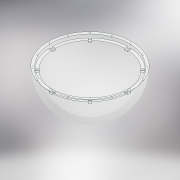
# Autodesk Inventor part: Bol
Saved by Autodesk Inventor 2022 (Build 260153000, 153)
## iProperties
Created: 2022-03-08
Part Number: Bol
Material: Glass
Document SubType Name: Modeling
Designer: 32497
Density: 2.18 g/cm^3
Appearance: Clear
Author: 32497
Autodesk Inventor part; units mm, degrees
ref_plane "YZ Plane" through (0, 0, 0) normal (1, 0, 0) x (0, 1, 0)
ref_plane "XZ Plane" through (0, 0, 0) normal (0, 1, 0) x (-1, 0, 0)
ref_plane "XY Plane" through (0, 0, 0) normal (0, 0, 1) x (1, 0, 0)
sketch "Sketch1" plane through (0, 0, 0) normal (0, 1, 0) x (-1, 0, 0)
  arc A0 (0, 150) -> (0, -150) centre (0, 0) ccw
  arc A1 (0, 130) -> (0, -130) centre (0, 0) ccw
  line L0 (0, -150) -> (0, 150)
  line L1 (150, 0) -> (-150, 0)
  circle A2 centre (0, 0) radius 141
  dimension "d0" = 300
  dimension "d1" = 260
  dimension "d9" = 282
  constraints: 5 point on circle, 4 end point, 3 centre point, 3 coincident, 2 point on line, 1 vertical
  measures "d0" diameter of A0
  measures "d1" diameter of A1
  measures "d9" diameter of A2
revolve "Revolution1" add sketch "Sketch1" angle 180 about axis through (0, 0, -150) along (0, 0, -1) contours L0 A2 L1 A0 | L1 A2 L0 A0 | L0 A1 L1 A2 | L1 A1 L0 A2
sketch "Sketch6" plane through (0, 0, 0) normal (0, 1, 0) x (1, 0, 0)
  circle A0 centre (0, 0) radius 140
  circle A1 centre (0, 0) radius 128.5
  dimension "d19" = 280
  dimension "d20" = 257
  constraints: 2 centre point, 2 coincident
  measures "d19" diameter of A0
  measures "d20" diameter of A1
extrude "Extrusion3" cut sketch "Sketch6" against normal blind 12.5
sketch "Sketch7" plane through (0, -12.5, 0) normal (0, 1, 0) x (1, 0, 0)
  line L0 (-5, 140.4975) -> (5, 140.4975)
  line L1 (5, 140.4975) -> (5, 128.8975)
  line L2 (5, 128.8975) -> (-5, 128.8975)
  line L3 (-5, 128.8975) -> (-5, 140.4975)
  circle A0 centre (0, 0) radius 129.3976 projected
  arc A1 (-5, 129.301) -> (0, 129.3976) centre (0, 0) ccw
  circle A2 centre (0, 0) radius 140 projected
  arc A3 (-5, 139.9107) -> (0, 140) centre (0, 0) ccw
  point P0 (5, 139.9107)
  point P1 (5, 129.301)
  dimension "d23" = 10
  dimension "d24" = 11.6
  dimension "d25" = 5
  dimension "d26" = 128.8975
  constraints: 8 end point, 8 point on circle, 2 centre point, 2 parallel, 2 point on line, 1 horizontal, 1 perpendicular
  measures "d23" distance of L1.end L2.end
  measures "d24" distance of L0.end L1.end
  measures "d25" distance from line of point (0, 0) L3
  measures "d26" distance from line of point (0, 0) L2
extrude "Extrusion4" cut sketch "Sketch7" against normal blind 5 contours A2 L1 A0 L3 | A0 L1 L2 L3 picked at (4.4446, 132.8554) picked at (0, 129.0642)
pattern_circular "Circular Pattern1" count 8 over 360 about axis through (0, -10, 0) along (0, 1, 0) of "Extrusion4"
sketch "Sketch8" plane through (0, 0, 0) normal (0, 1, 0) x (1, 0, 0)
  circle A0 centre (0, 145) radius 1
  circle A1 centre (0, 0) radius 150 projected
  dimension "d32" = 2
  dimension "d33" = 145
  constraints: 1 centre point
  measures "d32" diameter of A0
  measures "d33" distance of A1.centre A0.centre
extrude "Extrusion5" cut sketch "Sketch8" against normal blind 7 contours A0
pattern_circular "Circular Pattern2" count 16 over 360 about axis through (0, -10, 0) along (0, 1, 0) of "Extrusion5"
body "Solid1"
